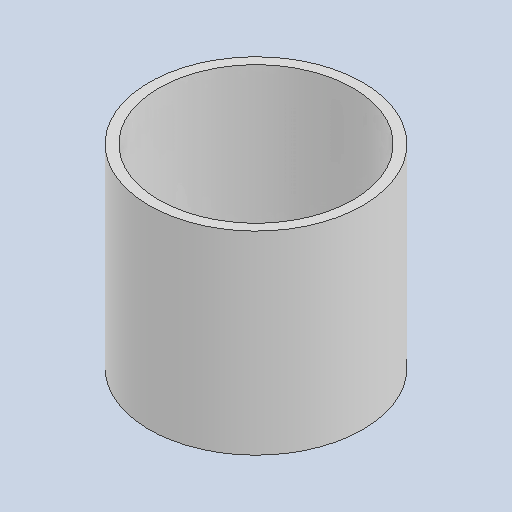
# Autodesk Inventor part: casing_cylindrical
Saved by Autodesk Inventor 2025 (Build 290162000, 162)
## iProperties
Created: 2026-08-03
Part Number: casing_cylindrical
Material: Ogólny
Document SubType Name: Modeling
Designer: zzapa
Density: 1 g/cm^3
Appearance: Domyślna
Author: zzapa
Autodesk Inventor part; units mm, degrees
ref_plane "YZ Plane" through (0, 0, 0) normal (1, 0, 0) x (0, 1, 0)
ref_plane "XZ Plane" through (0, 0, 0) normal (0, 1, 0) x (-1, 0, 0)
ref_plane "XY Plane" through (0, 0, 0) normal (0, 0, 1) x (1, 0, 0)
sketch "Szkic1" plane through (0, 0, 0) normal (0, 0, 1) x (1, 0, 0)
  line L0 (-7, 0) -> (42, 0) projected
  line L1 (33, 60) -> (30, 60)
  line L2 (30, 60) -> (30, 0)
  line L3 (30, 0) -> (33, 0)
  line L4 (33, 0) -> (33, 60)
  line L5 (0, -12) -> (0, 72) projected
  point P0 (0, 0)
  point P1 (30, 0)
  point P2 (33, 0)
  dimension "d0" = 30
  dimension "d1" = 3
  dimension "d2" = 60
  constraints: 8 end point, 2 parallel, 1 collinear, 1 horizontal, 1 perpendicular
  measures "d0" distance from line of point (0, 0) L2
  measures "d1" distance of L1.start L1.end
  measures "d2" distance of L3.end L1.start
revolve "Obrót1" add sketch "Szkic1" angle 360 about axis through (0, -10, 0) along (0, 1, 0)
equation "\"d0\" = casing_r_in"
equation "\"d1\" = casing_d"
equation "\"d2\" = casing_h"
equation "\"stator_out_d\" = 2.5"
equation "\"stator_h\" = 35"
equation "\"mag_size_x\" = 7"
equation "\"mag_size_y\" = 3"
equation "\"mag_corner_r\" = 0.4"
equation "\"magnet_ring_r\" = 27.5"
equation "\"magnet_ring_d\" = 3.3"
equation "\"magnet_ring_h\" = 36"
equation "\"magnet_ring_pocket_mag_size_x\" = 7.1"
equation "\"magnet_ring_pocket_mag_size_y\" = 3.1"
equation "\"magnet_ring_pocket_mag_size_z\" = 10.3"
equation "\"magnet_ring_pocket_radial_cut\" = 1.4"
equation "\"casing_h\" = 60"
equation "\"casing_d\" = 3"
equation "\"casing_r_in\" = 30"
equation "\"rotor_core_r\" = 15"
equation "\"coil_groove_ang\" = 18"
equation "\"rotor_out_r\" = 23"
equation "\"rotor_coil_groove_in_r\" = 17"
equation "\"rotor_coil_groove_ang\" = 18deg"
equation "\"rotor_coil_groove_in_correction_r\" = 18"
equation "\"rotor_plastic_h\" = 32"
equation "\"rotor_teeth_d\" = 1.5"
equation "\"shaft_d\" = 8"
equation "\"insert25m_d\" = 2.9"
equation "\"insert25m_corner\" = 0.5"
equation "\"insert25m_h\" = 7"
equation "\"rotor_plastic_insert_r\" = 37"
equation "\"shaft_lock_1_d\" = 8"
equation "\"shaf_lock_1_D\" = 32"
equation "\"shaft_lock_1_D\" = 44"
equation "\"shaft_lock_1_h1\" = 3.5"
equation "\"shaft_lock_1_insert_part_h\" = 8"
equation "\"shaft_lock_1_corner\" = 2"
equation "\"shaft_lock_1_insert_part_a\" = 18"
equation "\"shaft_lock_2_h1\" = 3.5"
equation "\"shaft_lock_2_d\" = 8"
equation "\"shaft_lock_2_insert_part_a\" = 18"
equation "\"shaft_lock_2_D\" = 44"
equation "\"shaft_lock_2_corner\" = 2"
equation "\"shaft_lock_2_insert_part_h\" = 7"
equation "\"shaft_lock_2_rotor_insert_grove_d_in\" = 36"
equation "\"shaft_lock_2_rotor_insert_grove_width_out\" = 5.5"
equation "\"shaft_lock_2_rotor_insert_grove_width_in\" = 7.6"
equation "\"shaft_lock_2_rotor_insert_r\" = 37"
equation "\"shaft_lock_2_rotor_insert_screw_d\" = 2.6"
equation "\"insert25m_pocket_d\" = 2.6"
equation "\"insert25m_pocket_D\" = 4.5"
equation "\"insert25m_pocket_nut_h\" = 1.5"
equation "\"insert_m2_pocket_d\" = 2.6"
equation "\"insert_m2_h\" = 7"
equation "\"insert_m2_d\" = 2.9"
equation "\"insert_m2_corner\" = 0.5"
equation "\"insert_m2_pocket_D\" = 4.5"
equation "\"insert_m2_pocket_nut_h\" = 1.5"
equation "\"shaft_lock_1_insert_part_corner\" = 6"
equation "\"shaft_lock_1_insert_part_pos\" = 4"
equation "\"shaft_lock_1_rotor_insert_grove_width_in\" = 7.6"
equation "\"shaft_lock_1_rotor_insert_r\" = 37"
equation "\"shaft_lock_1_rotor_insert_grove_d_in\" = 36"
equation "\"shaft_lock_1_rotor_insert_grove_width_out\" = 5.5"
equation "\"shaft_lock_1_shaft_insert_axial_cut_out_width\" = 12"
equation "\"shaft_lock_1_shaft_insert_axial_cut_in_width\" = 5.4"
equation "\"shaft_lock_1_shaft_insert_corner\" = 2"
equation "\"shaft_lock_1_shaft_insert_corner_finish\" = 0.5"
equation "\"shaft_lock_1_shaft_insert_pos\" = 2.5"
equation "\"shaft_lock_2_shaft_insert_corner\" = 2"
equation "\"shaft_lock_2_shaft_insert_pos\" = 2.5"
equation "\"shaft_lock_2_shaft_insert_axial_cut_in_width\" = 5.4"
equation "\"shaft_lock_2_shaft_insert_axial_cut_out_width\" = 12"
equation "\"shaft_lock_2_shaft_insert_corner_finish\" = 0.5"
